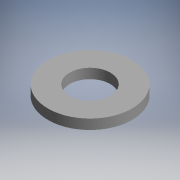
# Autodesk Inventor part: HCBST8washer2
Saved by Autodesk Inventor 2017.3 (Build 213256000, 256)
## iProperties
Part Number: HCBST8washer2
Material: Generic
Catalog Web Link: www.cadenas.de
Description: HCBSTw2-Washer Assembled Hexagon Socket Head Cap Screws
Vendor: MISUMI
Document SubType Name: Modeling
Designer: partserver
Manufacturer: MISUMI
Mass: 0.34834 g
Surface Area: 5.06676 cm^2
Volume: 0.34834 cm^3
Density: 1 g/cm^3
Appearance: PSOLRGB-192-192-192
Category: PARTsolutions
Company: MISUMI
Title: HCBST8
Author: Cadenas PARTsolutions
Comments: Washer Assembled Hexagon Socket Head Cap Screws
PSOL_IDENT_0: {$CADENAS_DATA\23d-libs\misumi\metric\38_al_extrusions_blackets\nuts\hcbst_washer.prj},161 {VTYP=3D}
PSOL_IDENT_1: ,{NB=HCBST8washer2},{LINA=HCBST8},{NN=HCBSTw2},{DATE=17.06.2021 07:12:01},{GEOMDATE=18.08.2009 10:36
PSOL_IDENT_2: :00},{VERSION=},{LINEID=110},{WBVAR=},{WBNUMERIC=}  {NB=HCBST8washer2},{LINA=HCBST8},{KT=DUMMY},{PN=
PSOL_IDENT_3: HCBST8},{M=8},{M1=8},{MP=8x1.25},{P=1.250},{C=14.5},{D=17.0},{AA=8.4},{DD=8.2},{TT=2.0}
NB: HCBST8washer2
NN: HCBSTw2
NT: Washer Assembled Hexagon Socket Head Cap Screws
NBSYN: $PN.washer2
LINA: HCBST8
CATALOG: Misumi
PN: HCBST8
M: 8
M1: 8
MP: 8x1.25
P: 1.25
C: 14.5
D: 17
AA: 8.4
DD: 8.2
TT: 2
SUPPLIER: MISUMI
ARTICLENO: HCBST8washer2
BOMINFO: HCBST8
CREATOR: CADENAS GmbH
Autodesk Inventor part; units mm, degrees
sketch "Sketch_2" plane through (0, 0, 0) normal (0, 0, 1) x (1, 0, 0)
  circle A0 centre (0, 0) radius 8.5
  circle A1 centre (0, 0) radius 4.1
  constraints: 2 centre point
extrude "Extrusion1" add sketch "Sketch_2" against normal blind 2
ref_plane "washer_to_bolt_XY" through (0, 0, 0) normal (0, 0, 1) x (1, 0, 0)
ref_plane "washer_to_bolt_YZ" through (0, 0, 0) normal (1, 0, 0) x (0, 1, 0)
ref_plane "washer_to_bolt_ZX" through (0, 0, 0) normal (0, 1, 0) x (0, 0, 1)
body "Solid1"
